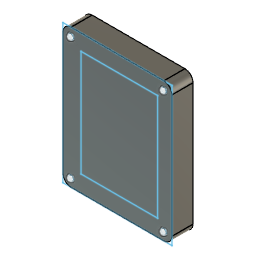
final (Autodesk Fusion 360 archive; units mm, degrees)
design "base_01_new"
part number: 2026-02-07-20-27-30-658
Autodesk Fusion 360 part; units mm, degrees
sketch "Sketch1" plane through (0, 0, 0) normal (0, 1, 0) x (1, 0, 0)
  line L0 (-90, -80) -> (-42.86, -80)
  line L1 (-42.86, -80) -> (-42.86, -14.63)
  line L2 (-42.86, -14.63) -> (-90, -14.63)
  line L3 (-90, -14.63) -> (-90, -80)
  line L4 (-34.1091, -89.705) -> (-101.2491, -89.705)
  line L5 (-101.2491, -89.705) -> (-101.2491, -4.335)
  line L6 (-101.2491, -4.335) -> (-34.1091, -4.335)
  line L7 (-34.1091, -4.335) -> (-34.1091, -89.705)
  circle A0 centre (-96.2491, -84.705) radius 1.45
  circle A1 centre (-39.1091, -84.705) radius 1.45
  circle A2 centre (-39.1091, -9.335) radius 1.45
  circle A3 centre (-96.2491, -9.335) radius 1.45
  dimension "d1" = 65.37
  dimension "d2" = 47.14
  dimension "d3" = 85.37
  dimension "d4" = 67.14
  dimension "d5" = 2.9
  dimension "d6" = 5
  dimension "d7" = 5
  dimension "d8" = 2.9
  dimension "d9" = 5
  dimension "d10" = 5
  dimension "d11" = 2.9
  dimension "d12" = 5
  dimension "d13" = 5
  dimension "d14" = 2.9
  dimension "d15" = 5
  dimension "d16" = 5
  constraint horizontal L0
  constraint vertical L1
  constraint horizontal L2
  constraint vertical L3
  constraint horizontal L4
  constraint vertical L5
  constraint horizontal L6
  constraint vertical L7
  measures "d1" distance of L0.start L2.end
  measures "d2" distance of L1 L3
  measures "d3" distance of L4.start L6.end
  measures "d4" distance of L5 L7
  measures "d5" diameter of A0
  measures "d6" distance of L5 A0.centre
  measures "d7" distance of L4 A0.centre
  measures "d8" diameter of A1
  measures "d9" distance of L7 A1.centre
  measures "d10" distance of L4 A1.centre
  measures "d11" diameter of A2
  measures "d12" distance of L6 A2.centre
  measures "d13" distance of L7 A2.centre
  measures "d14" diameter of A3
  measures "d15" distance of L5 A3.centre
  measures "d16" distance of L6 A3.centre
sketch "Sketch2" plane through (0, 0, 0) normal (0, 1, 0) x (1, 0, 0)
sketch "Sketch3" plane through (0, 0, 0) normal (0, 1, 0) x (1, 0, 0)
extrude "Extrude1" add sketch "Sketch1" along normal blind 13
extrude "Extrude2" add sketch "Sketch1" along normal blind 3 contours L0 L1 L2 L3
fillet "Fillet1" radius 5 1 edges at (-101.2491, 6.5, 89.705)
fillet "Fillet2" radius 5 1 edges at (-101.2491, 6.5, 4.335)
fillet "Fillet3" radius 5 1 edges at (-34.1091, 6.5, 4.335)
fillet "Fillet4" radius 5 1 edges at (-34.1091, 6.5, 89.705)

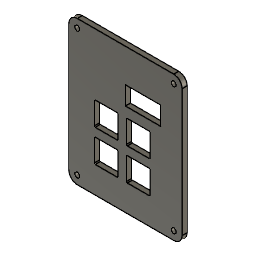
design "case_up_new"
part number: 2026-02-07-21-05-02-907
Autodesk Fusion 360 part; units mm, degrees
sketch "Sketch1" plane through (0, 0, 0) normal (0, 1, 0) x (1, 0, 0)
  line L0 (-60.7538, -33.1552) -> (6.3862, -33.1552)
  line L1 (6.3862, -33.1552) -> (6.3862, 52.2148)
  line L2 (6.3862, 52.2148) -> (-60.7538, 52.2148)
  line L3 (-60.7538, 52.2148) -> (-60.7538, -33.1552)
  line L4 (-50.7538, -23.1552) -> (-3.6138, -23.1552)
  line L5 (-3.6138, -23.1552) -> (-3.6138, 42.2148)
  line L6 (-3.6138, 42.2148) -> (-50.7538, 42.2148)
  line L7 (-50.7538, 42.2148) -> (-50.7538, -23.1552)
  line L8 (-50.747, 42.1269) -> (-12.647, 42.1269)
  line L9 (-50.747, 4.0269) -> (-50.747, 42.1269)
  line L10 (-45.133, 36.4505) -> (-32.133, 36.4505)
  line L11 (-45.133, 22.4505) -> (-32.133, 22.4505)
  line L12 (-45.633, 35.9505) -> (-45.633, 22.9505)
  line L13 (-31.633, 35.9505) -> (-31.633, 22.9505)
  arc A0 (-45.133, 36.4505) -> (-45.633, 35.9505) centre (-45.133, 35.9505) ccw
  arc A1 (-31.633, 35.9505) -> (-32.133, 36.4505) centre (-32.133, 35.9505) ccw
  arc A2 (-45.633, 22.9505) -> (-45.133, 22.4505) centre (-45.133, 22.9505) ccw
  arc A3 (-32.133, 22.4505) -> (-31.633, 22.9505) centre (-32.133, 22.9505) ccw
  line L14 (-26.083, 36.4505) -> (-13.083, 36.4505)
  line L15 (-26.083, 22.4505) -> (-13.083, 22.4505)
  line L16 (-26.583, 35.9505) -> (-26.583, 22.9505)
  line L17 (-12.583, 35.9505) -> (-12.583, 22.9505)
  arc A4 (-26.083, 36.4505) -> (-26.583, 35.9505) centre (-26.083, 35.9505) ccw
  arc A5 (-12.583, 35.9505) -> (-13.083, 36.4505) centre (-13.083, 35.9505) ccw
  arc A6 (-26.583, 22.9505) -> (-26.083, 22.4505) centre (-26.083, 22.9505) ccw
  arc A7 (-13.083, 22.4505) -> (-12.583, 22.9505) centre (-13.083, 22.9505) ccw
  line L18 (-45.133, 17.4005) -> (-32.133, 17.4005)
  line L19 (-45.133, 3.4005) -> (-32.133, 3.4005)
  line L20 (-45.633, 16.9005) -> (-45.633, 3.9005)
  line L21 (-31.633, 16.9005) -> (-31.633, 3.9005)
  arc A8 (-45.133, 17.4005) -> (-45.633, 16.9005) centre (-45.133, 16.9005) ccw
  arc A9 (-31.633, 16.9005) -> (-32.133, 17.4005) centre (-32.133, 16.9005) ccw
  arc A10 (-45.633, 3.9005) -> (-45.133, 3.4005) centre (-45.133, 3.9005) ccw
  arc A11 (-32.133, 3.4005) -> (-31.633, 3.9005) centre (-32.133, 3.9005) ccw
  line L22 (-26.083, 17.4005) -> (-13.083, 17.4005)
  line L23 (-26.083, 3.4005) -> (-13.083, 3.4005)
  line L24 (-26.583, 16.9005) -> (-26.583, 3.9005)
  line L25 (-12.583, 16.9005) -> (-12.583, 3.9005)
  arc A12 (-26.083, 17.4005) -> (-26.583, 16.9005) centre (-26.083, 16.9005) ccw
  arc A13 (-12.583, 16.9005) -> (-13.083, 17.4005) centre (-13.083, 16.9005) ccw
  arc A14 (-26.583, 3.9005) -> (-26.083, 3.4005) centre (-26.083, 3.9005) ccw
  arc A15 (-13.083, 3.4005) -> (-12.583, 3.9005) centre (-13.083, 3.9005) ccw
  line L26 (-48.158, 0.8755) -> (-10.058, 0.8755)
  line L27 (-48.158, 38.9755) -> (-10.058, 38.9755)
  line L28 (-48.158, 0.8755) -> (-48.158, 38.9755)
  line L29 (-10.058, 0.8755) -> (-10.058, 38.9755)
  circle A16 centre (1.3862, -28.1552) radius 1.45
  circle A17 centre (1.3862, 47.2148) radius 1.45
  circle A18 centre (-55.7538, 47.2148) radius 1.45
  circle A19 centre (-55.7538, -28.1552) radius 1.45
  line L30 (-6.4728, -13.3522) -> (-27.2128, -13.3522)
  line L31 (-27.2128, -13.3522) -> (-27.2128, -2.4922)
  line L32 (-27.2128, -2.4922) -> (-6.4728, -2.4922)
  line L33 (-6.4728, -2.4922) -> (-6.4728, -13.3522)
  dimension "d1" = 85.37
  dimension "d2" = 67.14
  dimension "d3" = 10
  dimension "d4" = 10
  dimension "d5" = 10
  dimension "d6" = 10
  dimension "d12" = 2.9
  dimension "d13" = 5
  dimension "d14" = 5
  dimension "d15" = 2.9
  dimension "d16" = 5
  dimension "d17" = 5
  dimension "d18" = 2.9
  dimension "d19" = 5
  dimension "d20" = 5
  dimension "d21" = 2.9
  dimension "d22" = 5
  dimension "d23" = 5
  dimension "d28" = 10.86
  dimension "d29" = 20.74
  dimension "d30" = 2.859
  dimension "d31" = 9.803
  constraint horizontal L0
  constraint vertical L1
  constraint horizontal L2
  constraint vertical L3
  constraint horizontal L4
  constraint vertical L5
  constraint horizontal L6
  constraint vertical L7
  constraint horizontal L30
  constraint vertical L31
  constraint horizontal L32
  constraint vertical L33
  measures "d1" distance of L0.start L2.end
  measures "d2" distance of L1 L3
  measures "d3" distance of L1 L5
  measures "d4" distance of L2 L6
  measures "d5" distance of L0 L4
  measures "d6" distance of L3 L7
  measures "d12" diameter of A16
  measures "d13" distance of L1 A16.centre
  measures "d14" distance of L0 A16.centre
  measures "d15" diameter of A17
  measures "d16" distance of L1 A17.centre
  measures "d17" distance of L2 A17.centre
  measures "d18" diameter of A18
  measures "d19" distance of L2 A18.centre
  measures "d20" distance of L3 A18.centre
  measures "d21" diameter of A19
  measures "d22" distance of L0 A19.centre
  measures "d23" distance of L3 A19.centre
  measures "d28" distance of L30.start L32.end
  measures "d29" distance of L31 L33
  measures "d30" distance of L5 L33
  measures "d31" distance of L4 L30
extrude "Extrude1" add sketch "Sketch1" along normal blind 3 contours L0 L1 L2 L3 | L4 L5 L6 L7 | L26 L27 L28 L29
fillet "Fillet1" radius 5 4 edges at (6.3862, 1.5, -52.2148) (6.3862, 1.5, 33.1552) (-60.7538, 1.5, 33.1552) (-60.7538, 1.5, -52.2148)
